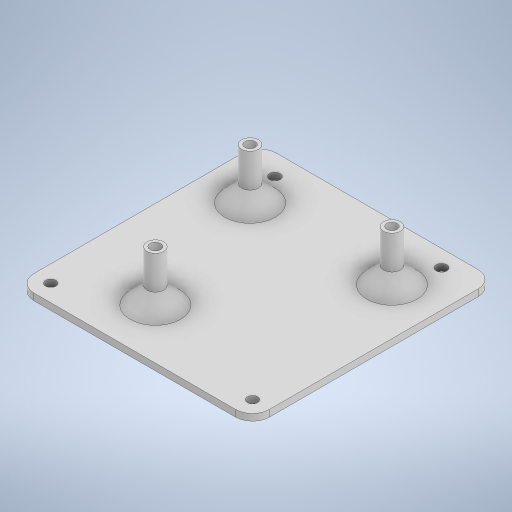
# Autodesk Inventor part: SimpleRTK - PlateAdapter
Saved by Autodesk Inventor 2023 (Build 270158000, 158)
## iProperties
Created: 2023-01-25
Part Number: SimpleRTK - PlateAdapter
Material: Generic
Document SubType Name: Modeling
Designer: Administrator
Density: 1 g/cm^3
Appearance: Default
Author: Administrator
Autodesk Inventor part; units mm, degrees
ref_plane "YZ Plane" through (0, 0, 0) normal (1, 0, 0) x (0, 1, 0)
ref_plane "XZ Plane" through (0, 0, 0) normal (0, 1, 0) x (-1, 0, 0)
ref_plane "XY Plane" through (0, 0, 0) normal (0, 0, 1) x (1, 0, 0)
sketch "Sketch1" plane through (0, 0, 0) normal (0, 0, 1) x (1, 0, 0)
  circle A0 centre (8.9, 50.3645) radius 1.55
  circle A1 centre (8.9, 50.3645) radius 1.5
  circle A2 centre (51.1, 50.3645) radius 1.55
  circle A3 centre (51.1, 50.3645) radius 1.5
  circle A4 centre (60, 0) radius 1.55
  circle A5 centre (60, 0) radius 1.5
  circle A6 centre (0, 0) radius 1.55
  circle A7 centre (0, 0) radius 1.5
  circle A8 centre (54.13, 62.07) radius 1.5999
  circle A9 centre (5.87, 60.8) radius 1.5999
  circle A10 centre (21.11, 10) radius 1.5999
  circle A11 centre (54.13, 62.07) radius 1.5
  circle A12 centre (5.87, 60.8) radius 1.5
  circle A13 centre (21.11, 10) radius 1.5
  line L0 (-5, 67.07) -> (65, 67.07)
  line L1 (65, 67.07) -> (65, -5)
  line L2 (65, -5) -> (-5, -5)
  line L3 (-5, -5) -> (-5, 67.07)
  point P0 (17, 90.5)
  dimension "d0" = 3
  dimension "d1" = 3
  dimension "d2" = 3
  dimension "d3" = 3
  dimension "d4" = 8.9
  dimension "d5" = 8.9
  dimension "d6" = 42.2
  dimension "d7" = 50.3645
  dimension "d8" = 0
  dimension "d9" = 0
  dimension "d10" = 3
  dimension "d11" = 3
  dimension "d12" = 3
  dimension "d13" = 50.8
  dimension "d14" = 52.07
  dimension "d15" = 15.24
  dimension "d16" = 33.02
  dimension "d18" = 10
  dimension "d19" = 5.87
  dimension "d22" = 5
  dimension "d23" = 5
  dimension "d24" = 5
  dimension "d25" = 5
  constraints: 14 centre point, 8 end point, 7 coincident, 2 parallel, 1 horizontal, 1 perpendicular
  measures "d0" diameter of A1
  measures "d1" diameter of A3
  measures "d2" diameter of A5
  measures "d3" diameter of A7
  measures "d4" horizontal distance of point (0, 0) A1.centre
  measures "d5" horizontal distance of A5.centre A3.centre
  measures "d6" distance of A3.centre A1.centre
  measures "d7" vertical distance of point (0, 0) A1.centre
  measures "d8" vertical distance of point (0, 0) A5.centre
  measures "d9" vertical distance of A1.centre A3.centre
  measures "d10" diameter of A11
  measures "d11" diameter of A12
  measures "d12" diameter of A13
  measures "d13" vertical distance of A10.centre A9.centre
  measures "d14" vertical distance of A8.centre A10.centre
  measures "d15" horizontal distance of A10.centre A9.centre
  measures "d16" horizontal distance of A11.centre A10.centre
  measures "d18" vertical distance of A10.centre point (0, 0)
  measures "d19" horizontal distance of point (0, 0) A9.centre
  measures "d22" distance from line of A11.centre L0
  measures "d23" distance from line of A5.centre L2
  measures "d24" distance from line of L1 A5.centre
  measures "d25" distance from line of L3 point (0, 0)
extrude "Extrusion1" add sketch "Sketch1" along normal blind 2 contours L0 L1 L2 L3
fillet "Fillet1" radius 5 4 edges at (-5, -5, 1) (65, -5, 1) (65, 67.07, 1) (-5, 67.07, 1)
sketch "Sketch2" plane through (0, 0, 2) normal (0, 0, 1) x (1, 0, 0)
  circle A0 centre (8.9, 50.3645) radius 1.55 projected
  circle A1 centre (8.9, 50.3645) radius 2.5
  circle A2 centre (51.1, 50.3645) radius 1.55 projected
  circle A3 centre (51.1, 50.3645) radius 2.5
  circle A4 centre (21.11, 10) radius 1.5999 projected
  circle A5 centre (21.11, 10) radius 2.5
  point P0 (0, 0)
  dimension "d29" = 5
  dimension "d30" = 5
  dimension "d31" = 5
  constraints: 3 centre point, 3 coincident
  measures "d29" diameter of A1
  measures "d30" diameter of A3
  measures "d31" diameter of A5
extrude "Extrusion2" add sketch "Sketch2" along normal blind 15
chamfer "Chamfer1" distance 5 angle 45 3 edges at (18.61, 10, 2) (6.4, 50.3645, 2) (48.6, 50.3645, 2)
equation "\"d19\" = -0.5 * d16 - 0.5 * d15 + 0.5 * d6 + 0.5 * d5 + 0.5 * d4"
body "Solid1"
